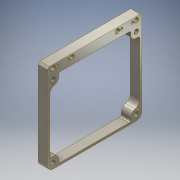
# Autodesk Inventor part: Корпус02
Saved by Autodesk Inventor 2016 (Build 200138000, 138)
## iProperties
Created: 2021-04-23
Part Number: Корпус02
Material: Типовые
Document SubType Name: Modeling
Designer: Лол
Density: 1 g/cm^3
Appearance: Титан — полированный
Author: Лол
Autodesk Inventor part; units mm, degrees
ref_plane "YZ Plane" through (0, 0, 0) normal (1, 0, 0) x (0, 1, 0)
ref_plane "XZ Plane" through (0, 0, 0) normal (0, 1, 0) x (-1, 0, 0)
ref_plane "XY Plane" through (0, 0, 0) normal (0, 0, 1) x (1, 0, 0)
sketch "Эскиз1" plane through (0, 0, 0) normal (0, 0, 1) x (1, 0, 0)
  line L0 (-12.5, 120) -> (12.5, 120)
  line L1 (12.5, 120) -> (12.5, -130)
  line L2 (12.5, -130) -> (-12.5, -130)
  line L3 (-12.5, -130) -> (-12.5, 120)
  line L4 (-17.5, 0) -> (17.5, 0) projected
  line L5 (0, -180) -> (0, 170) projected
  point P0 (0, 0)
  dimension "d0" = 250
  dimension "d1" = 25
  dimension "d2" = 120
  constraints: 8 end point, 2 parallel, 1 horizontal, 1 perpendicular, 1 other
  measures "d0" distance of L0.end L1.end
  measures "d1" distance of L0.start L0.end
  measures "d2" distance between parallel lines of L4 L0
extrude "Выдавливание1" add sketch "Эскиз1" along normal blind 100 and the other way blind 120
sketch "Эскиз2" plane through (12.5, -130, 100) normal (1, 0, 0) x (0, 0, -1)
  line L0 (0, 250) -> (220, 250) projected
  line L1 (0, 0) -> (0, 250) projected
  line L2 (220, 250) -> (220, 0) projected
  line L3 (0, 0) -> (220, 0) projected
  line L4 (6, 244) -> (214, 244)
  line L5 (214, 244) -> (214, 6)
  line L6 (214, 6) -> (6, 6)
  line L7 (6, 6) -> (6, 244)
  point P0 (100, 130)
  dimension "d7" = 6
  dimension "d8" = 6
  dimension "d9" = 6
  dimension "d10" = 6
  constraints: 8 end point, 2 parallel, 1 horizontal, 1 perpendicular
  measures "d7" distance between parallel lines of L0 L4
  measures "d8" distance between parallel lines of L2 L5
  measures "d9" distance between parallel lines of L3 L6
  measures "d10" distance between parallel lines of L1 L7
extrude "Выдавливание2" cut sketch "Эскиз2" against normal through all contours L4 L5 L6 L7
fillet "Сопряжение1" radius 15 4 edges at (0, 120, 100) (0, 120, -120) (0, -130, 100) (0, -130, -120)
sketch "Эскиз3" plane through (12.5, -115, -120) normal (1, 0, 0) x (0, 0, -1)
  arc A0 (-205, 235) -> (-220, 220) centre (-205, 220) ccw projected
  arc A1 (0, 220) -> (-15, 235) centre (-15, 220) ccw projected
  arc A2 (-15, -15) -> (0, 0) centre (-15, 0) ccw projected
  arc A3 (-220, 0) -> (-205, -15) centre (-205, 0) ccw projected
  arc A4 (-15, -15) -> (0, 0) centre (-15, 0) ccw projected
  circle A5 centre (-205, 0) radius 15
  circle A6 centre (-15, 0) radius 15
  circle A7 centre (-15, 220) radius 15
  circle A8 centre (-205, 220) radius 15
  point P0 (-120, 115)
  dimension "d15" = 30
  constraints: 4 centre point, 4 coincident, 3 equal radius
  measures "d15" diameter of A8
extrude "Выдавливание3" add sketch "Эскиз3" against normal up to surface (25 mm away)
fillet "Сопряжение2" radius 5 6 edges at (0, 93, 94) (0, 93, -114) (0, -103, -114) (0, -103, 94) (0, 114, 73) (0, -124, -93)
sketch "Эскиз4" plane through (-12.5, -115, -120) normal (-1, 0, 0) x (0, 0, 1)
  line L0 (0, 0) -> (0, 220) projected
  arc A0 (0, 0) -> (15, -15) centre (15, 0) ccw projected
  line L1 (205, -15) -> (15, -15) projected
  arc A1 (205, -15) -> (220, 0) centre (205, 0) ccw projected
  line L2 (220, 220) -> (220, 0) projected
  arc A2 (220, 220) -> (205, 235) centre (205, 220) ccw projected
  line L3 (15, 235) -> (205, 235) projected
  arc A3 (15, 235) -> (0, 220) centre (15, 220) ccw projected
  line L4 (27, 229) -> (185.4041, 229) projected
  arc A4 (190.3031, 223) -> (208, 205.3031) centre (205, 220) ccw projected
  arc A5 (214, 200.4041) -> (208, 205.3031) centre (209, 200.4041) ccw projected
  line L5 (214, 200.4041) -> (214, 19.5959) projected
  arc A6 (208, 14.6969) -> (214, 19.5959) centre (209, 19.5959) ccw projected
  arc A7 (208, 14.6969) -> (193, -9) centre (205, 0) ccw projected
  line L6 (193, -9) -> (34.5959, -9) projected
  arc A8 (29.6969, -3) -> (12, 14.6969) centre (15, 0) ccw projected
  arc A9 (6, 19.5959) -> (12, 14.6969) centre (11, 19.5959) ccw projected
  line L7 (6, 19.5959) -> (6, 200.4041) projected
  arc A10 (12, 205.3031) -> (6, 200.4041) centre (11, 200.4041) ccw projected
  arc A11 (12, 205.3031) -> (27, 229) centre (15, 220) ccw projected
  circle A12 centre (15, 0) radius 5.1
  circle A13 centre (15, 220) radius 5.1
  arc A14 (220, 220) -> (205, 235) centre (205, 220) ccw projected
  circle A15 centre (205, 220) radius 5.1
  circle A16 centre (205, 0) radius 5.1
  arc A17 (190.3031, 223) -> (185.4041, 229) centre (185.4041, 224) ccw projected
  arc A18 (29.6969, -3) -> (34.5959, -9) centre (34.5959, -4) ccw projected
  point P0 (120, 115)
  dimension "d19" = 10.2
  constraints: 4 centre point, 4 coincident, 3 equal radius
  measures "d19" diameter of A12
extrude "Выдавливание4" cut sketch "Эскиз4" against normal through all contours A12 | A13 | A15 | A16
fillet "Сопряжение4" radius 15 2 edges at (0, 114, -93) (0, -124, 73)
sketch "Эскиз6" plane through (-12.5, -115, -120) normal (-1, 0, 0) x (0, 0, 1)
  circle A0 centre (15, 220) radius 5.1 projected
  circle A1 centre (205, 0) radius 5.1 projected
  circle A2 centre (195, -5) radius 3
  circle A3 centre (25, 225) radius 3
  point P0 (120, 115)
  dimension "d35" = 6
  dimension "d37" = 10
  dimension "d38" = 5
  dimension "d39" = 230
  dimension "d40" = 170
  constraints: 2 centre point, 1 equal radius
  measures "d35" diameter of A3
  measures "d37" horizontal distance of A2.centre A1.centre
  measures "d38" vertical distance of A1.centre A2.centre
  measures "d39" vertical distance of A3.centre A2.centre
  measures "d40" horizontal distance of A3.centre A2.centre
extrude "Выдавливание6" cut sketch "Эскиз6" against normal through all contours A2 | A3
chamfer "Фаска2" distance 0.6 angle 45 4 edges at (-12.5, 110, -98) (-12.5, -120, 72) (12.5, -120, 72) (12.5, 110, -98)
sketch "Эскиз7" plane through (0, 0, 0) normal (1, 0, 0) x (0, 1, 0)
  line L0 (120, -105) -> (120, 85) projected
  line L1 (-130, 85) -> (-130, -105) projected
  arc A0 (105, -120) -> (120, -105) centre (105, -105) ccw projected
  arc A1 (105, -120) -> (120, -105) centre (105, -105) ccw
  arc A2 (-130, -105) -> (-115, -120) centre (-115, -105) ccw
  line L2 (105, -120) -> (-115, -120)
  line L3 (105, 100) -> (-115, 100) projected
  arc A3 (120, 85) -> (105, 100) centre (105, 85) ccw projected
  arc A4 (-115, 100) -> (-130, 85) centre (-115, 85) ccw projected
  arc A5 (120, 85) -> (105, 100) centre (105, 85) ccw
  arc A6 (-115, 100) -> (-130, 85) centre (-115, 85) ccw
  line L4 (120, 120) -> (-130, 120)
  line L5 (-130, 120) -> (-130, 85)
  line L6 (120, 120) -> (120, 85)
  point P0 (0, 0)
  dimension "d52" = 20
  constraints: 10 end point, 8 point on circle, 4 centre point, 4 coincident, 3 tangent, 2 concentric, 2 horizontal, 1 parallel, 1 perpendicular
  measures "d52" distance between parallel lines of L3 L4
extrude "Выдавливание7" add sketch "Эскиз7" along normal mid plane 25 contours A3 L3 A4 L5 L4 L6
chamfer "Фаска3" distance 5 angle 45 2 edges at (0, 120, 120) (0, -130, 120)
sketch "Эскиз8" plane through (0, 0, 0) normal (1, 0, 0) x (0, 1, 0)
  line L0 (-130, 115) -> (-130, -105) construction
  line L1 (120, -105) -> (120, 115) projected
  line L2 (-125, 120) -> (115, 120) projected
  line L3 (120, 115) -> (120, -105) projected
  line L4 (-130, 111) -> (120, 111) construction
  circle A0 centre (-115, 111) radius 5
  circle A1 centre (-65, 111) radius 5
  circle A2 centre (105, 111) radius 5
  circle A3 centre (55, 111) radius 5
  line L5 (-130, 115) -> (-130, -105) projected
  line L6 (115, 120) -> (-125, 120) projected
  line L7 (-130, 102) -> (-50, 102) construction
  line L8 (-50, 102) -> (-50, 120) construction
  line L9 (-50, 120) -> (-130, 120) construction
  line L10 (-130, 120) -> (-130, 102) construction
  circle A4 centre (-104, 111) radius 3
  circle A5 centre (-76, 111) radius 3
  circle A6 centre (66, 111) radius 3
  circle A7 centre (94, 111) radius 3
  point P0 (0, 0)
  dimension "d53" = 9
  dimension "d54" = 10
  dimension "d55" = 15
  dimension "d56" = 15
  dimension "d57" = 50
  dimension "d58" = 50
  dimension "d59" = 80
  dimension "d60" = 18
  dimension "d61" = 6
  dimension "d62" = 11
  dimension "d64" = 11
  dimension "d66" = 28
  dimension "d67" = 28
  constraints: 8 centre point, 8 end point, 6 equal radius, 4 point on line, 2 parallel, 1 horizontal, 1 perpendicular, 11 other
  measures "d54" diameter of A0
  measures "d55" distance from line of A0.centre L0
  measures "d56" distance from line of A2.centre L1
  measures "d57" distance of A1.centre A0.centre
  measures "d58" distance of A2.centre A3.centre
  measures "d59" distance of L7.start L7.end
  measures "d60" distance between parallel lines of L2 L7
  measures "d61" diameter of A4
  measures "d62" distance of A4.centre A0.centre
  measures "d64" distance of A3.centre A6.centre
  measures "d66" distance of A5.centre A4.centre
  measures "d67" distance of A7.centre A6.centre
hole "Отверстие1" at (0, -104, 111) at (0, -76, 111) at (0, 94, 111) at (0, 66, 111) direction (1, 0, 0) diameter 6 end through all
hole "Отверстие2" at (0, -115, 111) at (0, -65, 111) at (0, 55, 111) at (0, 105, 111) direction (1, 0, 0) diameter 10.5 depth 12.5 tip angle 118
hole "Отверстие3" at (0, -65, 111) at (0, 55, 111) at (0, 105, 111) at (0, -115, 111) direction (-1, 0, 0) diameter 10.5 end through all
hole "Отверстие4" at (0, -104, 111) at (0, -76, 111) at (0, 94, 111) at (0, 66, 111) direction (-1, 0, 0) diameter 6 end through all
chamfer "Фаска4" distance 1 angle 45 8 edges at (-12.5, -115, 116.25) (-12.5, -65, 116.25) (-12.5, 55, 116.25) (-12.5, 105, 116.25) (12.5, -115, 105.75) (12.5, -65, 105.75) (12.5, 55, 105.75) (12.5, 105, 105.75)
chamfer "Фаска5" distance 0.6 angle 45 8 edges at (12.5, 94, 108) (12.5, 66, 108) (12.5, -76, 108) (12.5, -104, 108) (-12.5, -104, 114) (-12.5, -76, 114) (-12.5, 94, 114) (-12.5, 66, 114)
chamfer "Фаска6" distance 1 angle 45 8 edges at (12.5, 105, -110.1) (12.5, -115, -110.1) (12.5, 105, 79.9) (12.5, -115, 79.9) (-12.5, -115, 79.9) (-12.5, 105, 79.9) (-12.5, 105, -110.1) (-12.5, -115, -110.1)
